Autodesk Fusion 360 part; units mm, degrees
note: some values were not read from the file. Set by a fixed rule: which sketch regions a step uses.
(part 26 of 59)
  spline S30 degree 5 poles (-12.6495, -13.6461) (-12.6495, -13.6462) (-12.6496, -13.6464) (-12.6497, -13.6467) (-12.65, -13.6471) (-12.6503, -13.6478) (-12.6506, -13.6486) (-12.651, -13.6495) (-12.6515, -13.6504) (-12.652, -13.6515) (-12.6526, -13.6527) (-12.6531, -13.654) (-12.6538, -13.6554) (-12.6544, -13.6569) (-12.6551, -13.6585) (-12.6559, -13.6602) (-12.6567, -13.6619) (-12.6575, -13.6638) (-12.6583, -13.6658) (-12.6592, -13.6678) (-12.6602, -13.67) (-12.6611, -13.6722) (-12.6621, -13.6745) (-12.6631, -13.6769) (-12.6642, -13.6794) (-12.6653, -13.682) (-12.6664, -13.6847) (-12.6676, -13.6874) (-12.6687, -13.6903) (-12.6699, -13.6932) (-12.6712, -13.6962) (-12.6724, -13.6993) (-12.6737, -13.7024) (-12.675, -13.7057) (-12.6764, -13.709) (-12.6778, -13.7124) (-12.6791, -13.7159) (-12.6806, -13.7195) (-12.682, -13.7231) (-12.6834, -13.7269) (-12.6849, -13.7307) (-12.6864, -13.7345) (-12.688, -13.7385) (-12.6895, -13.7425) (-12.6911, -13.7466) (-12.6927, -13.7508) (-12.6943, -13.755) (-12.6959, -13.7594) (-12.6975, -13.7638) (-12.6992, -13.7682) (-12.7009, -13.7728) (-12.7026, -13.7774) (-12.7043, -13.782) (-12.706, -13.7868) (-12.7077, -13.7916) (-12.7095, -13.7965) (-12.7113, -13.8015) (-12.7131, -13.8065) (-12.7149, -13.8116) (-12.7167, -13.8167) (-12.7185, -13.822) (-12.7204, -13.8273) (-12.7222, -13.8326) (-12.7241, -13.838) (-12.726, -13.8435) (-12.7279, -13.8491) (-12.7298, -13.8547) (-12.7317, -13.8604) (-12.7336, -13.8661) (-12.7356, -13.8719) (-12.7375, -13.8778) (-12.7395, -13.8837) (-12.7414, -13.8897) (-12.7434, -13.8958) (-12.7454, -13.9019) (-12.7474, -13.9081) (-12.7494, -13.9144) (-12.7514, -13.9207) (-12.7534, -13.927) (-12.7555, -13.9335) (-12.7575, -13.9399) (-12.7596, -13.9465) (-12.7616, -13.9531) (-12.7637, -13.9598) (-12.7657, -13.9665) (-12.7678, -13.9733) (-12.7699, -13.9801) (-12.772, -13.987) (-12.774, -13.9939) (-12.7761, -14.0009) (-12.7782, -14.008) (-12.7803, -14.0151) (-12.7824, -14.0223) (-12.7845, -14.0296) (-12.7867, -14.0368) (-12.7888, -14.0442) (-12.7909, -14.0516) (-12.793, -14.059) (-12.7952, -14.0665) (-12.7973, -14.0741) (-12.7994, -14.0817) (-12.8016, -14.0894) (-12.8037, -14.0971) (-12.8058, -14.1049) (-12.808, -14.1127) (-12.8101, -14.1206) (-12.8123, -14.1286) (-12.8144, -14.1365) (-12.8166, -14.1446) (-12.8187, -14.1527) (-12.8208, -14.1608) (-12.823, -14.169) (-12.8251, -14.1773) (-12.8273, -14.1856) (-12.8294, -14.1939) (-12.8316, -14.2023) (-12.8337, -14.2108) (-12.8359, -14.2193) (-12.838, -14.2278) (-12.8402, -14.2364) (-12.8423, -14.2451) (-12.8445, -14.2537) (-12.8466, -14.2625) (-12.8487, -14.2713) (-12.8509, -14.2801) (-12.853, -14.289) (-12.8551, -14.298) (-12.8573, -14.3069) (-12.8594, -14.316) (-12.8615, -14.3251) (-12.8636, -14.3342) (-12.8658, -14.3434) (-12.8679, -14.3526) (-12.87, -14.3619) (-12.8721, -14.3712) (-12.8742, -14.3806) (-12.8763, -14.39) (-12.8784, -14.3994) (-12.8805, -14.4089) (-12.8826, -14.4185) (-12.8847, -14.4281) (-12.8867, -14.4377) (-12.8888, -14.4474) (-12.8909, -14.4571) (-12.8929, -14.4669) (-12.895, -14.4767) (-12.8971, -14.4866) (-12.8991, -14.4965) (-12.9011, -14.5064) (-12.9032, -14.5164) (-12.9052, -14.5265) (-12.9072, -14.5365) (-12.9093, -14.5467) (-12.9113, -14.5568) (-12.9133, -14.5671) (-12.9153, -14.5773) (-12.9173, -14.5876) (-12.9193, -14.5979) (-12.9213, -14.6083) (-12.9232, -14.6188) (-12.9252, -14.6292) (-12.9272, -14.6397) (-12.9291, -14.6503) (-12.9311, -14.6609) (-12.933, -14.6715) (-12.9349, -14.6822) (-12.9368, -14.6929) (-12.9388, -14.7037) (-12.9407, -14.7145) (-12.9426, -14.7253) (-12.9445, -14.7362) (-12.9463, -14.7471) (-12.9482, -14.7581) (-12.9501, -14.7691) (-12.9519, -14.7801) (-12.9538, -14.7912) (-12.9556, -14.8023) (-12.9574, -14.8135) (-12.9593, -14.8247) (-12.9611, -14.8359) (-12.9629, -14.8472) (-12.9647, -14.8585) (-12.9665, -14.8699) (-12.9682, -14.8813) (-12.97, -14.8927) (-12.9718, -14.9042) (-12.9735, -14.9157) (-12.9752, -14.9273) (-12.977, -14.9388) (-12.9787, -14.9505) (-12.9804, -14.9621) (-12.9821, -14.9738) (-12.9838, -14.9856) (-12.9854, -14.9974) (-12.9871, -15.0092) (-12.9887, -15.021) (-12.9904, -15.0329) (-12.992, -15.0449) (-12.9936, -15.0568) (-12.9952, -15.0688) (-12.9968, -15.0809) (-12.9984, -15.0929) (-13, -15.105) (-13.0016, -15.1172) (-13.0031, -15.1294) (-13.0047, -15.1416) (-13.0062, -15.1539) (-13.0077, -15.1661) (-13.0092, -15.1785) (-13.0107, -15.1908) (-13.0122, -15.2032) (-13.0136, -15.2157) (-13.0151, -15.2281) (-13.0165, -15.2406) (-13.018, -15.2532) (-13.0194, -15.2658) (-13.0208, -15.2784) (-13.0222, -15.291) (-13.0236, -15.3037) (-13.0249, -15.3164) (-13.0263, -15.3291) (-13.0276, -15.3419) (-13.029, -15.3547) (-13.0303, -15.3676) (-13.0316, -15.3805) (-13.0329, -15.3934) (-13.0342, -15.4063) (-13.0354, -15.4193) (-13.0367, -15.4323) (-13.0379, -15.4454) (-13.0391, -15.4585) (-13.0404, -15.4716) (-13.0415, -15.4848) (-13.0427, -15.4979) (-13.0439, -15.5112) (-13.0451, -15.5244) (-13.0462, -15.5377) (-13.0473, -15.551) (-13.0484, -15.5644) (-13.0495, -15.5777) (-13.0506, -15.5911) (-13.0515, -15.6019) (-13.0521, -15.61) (-13.0525, -15.6154) (-13.0527, -15.6181) knots 0 0 0 0 0 0 0.00416667 0.00833333 0.0125 0.01666667 0.02083333 0.025 0.02916667 0.03333333 0.0375 0.04166667 0.04583333 0.05 0.05416667 0.05833333 0.0625 0.06666667 0.07083333 0.075 0.07916667 0.08333333 0.0875 0.09166667 0.09583333 0.1 0.10416667 0.10833333 0.1125 0.11666667 0.12083333 0.125 0.12916667 0.13333333 0.1375 0.14166667 0.14583333 0.15 0.15416667 0.15833333 0.1625 0.16666667 0.17083333 0.175 0.17916667 0.18333333 0.1875 0.19166667 0.19583333 0.2 0.20416667 0.20833333 0.2125 0.21666667 0.22083333 0.225 0.22916667 0.23333333 0.2375 0.24166667 0.24583333 0.25 0.25416667 0.25833333 0.2625 0.26666667 0.27083333 0.275 0.27916667 0.28333333 0.2875 0.29166667 0.29583333 0.3 0.30416667 0.30833333 0.3125 0.31666667 0.32083333 0.325 0.32916667 0.33333333 0.3375 0.34166667 0.34583333 0.35 0.35416667 0.35833333 0.3625 0.36666667 0.37083333 0.375 0.37916667 0.38333333 0.3875 0.39166667 0.39583333 0.4 0.40416667 0.40833333 0.4125 0.41666667 0.42083333 0.425 0.42916667 0.43333333 0.4375 0.44166667 0.44583333 0.45 0.45416667 0.45833333 0.4625 0.46666667 0.47083333 0.475 0.47916667 0.48333333 0.4875 0.49166667 0.49583333 0.5 0.50416667 0.50833333 0.5125 0.51666667 0.52083333 0.525 0.52916667 0.53333333 0.5375 0.54166667 0.54583333 0.55 0.55416667 0.55833333 0.5625 0.56666667 0.57083333 0.575 0.57916667 0.58333333 0.5875 0.59166667 0.59583333 0.6 0.60416667 0.60833333 0.6125 0.61666667 0.62083333 0.625 0.62916667 0.63333333 0.6375 0.64166667 0.64583333 0.65 0.65416667 0.65833333 0.6625 0.66666667 0.67083333 0.675 0.67916667 0.68333333 0.6875 0.69166667 0.69583333 0.7 0.70416667 0.70833333 0.7125 0.71666667 0.72083333 0.725 0.72916667 0.73333333 0.7375 0.74166667 0.74583333 0.75 0.75416667 0.75833333 0.7625 0.76666667 0.77083333 0.775 0.77916667 0.78333333 0.7875 0.79166667 0.79583333 0.8 0.80416667 0.80833333 0.8125 0.81666667 0.82083333 0.825 0.82916667 0.83333333 0.8375 0.84166667 0.84583333 0.85 0.85416667 0.85833333 0.8625 0.86666667 0.87083333 0.875 0.87916667 0.88333333 0.8875 0.89166667 0.89583333 0.9 0.90416667 0.90833333 0.9125 0.91666667 0.92083333 0.925 0.92916667 0.93333333 0.9375 0.94166667 0.94583333 0.95 0.95416667 0.95833333 0.9625 0.96666667 0.97083333 0.975 0.97916667 0.98333333 0.9875 0.99166667 0.99583333 1 1 1 1 1 1
  arc A39 (-13.0527, -15.6181) -> (-12.1618, -16.0147) centre (0, 12.5) ccw
  spline S31 degree 5 poles (-12.1618, -16.0147) (-12.16, -16.0128) (-12.1562, -16.0089) (-12.1506, -16.003) (-12.1432, -15.9951) (-12.134, -15.9854) (-12.1248, -15.9756) (-12.1156, -15.9658) (-12.1065, -15.9561) (-12.0973, -15.9464) (-12.0883, -15.9366) (-12.0792, -15.9269) (-12.0702, -15.9172) (-12.0613, -15.9075) (-12.0523, -15.8978) (-12.0434, -15.8882) (-12.0345, -15.8785) (-12.0257, -15.8689) (-12.0169, -15.8593) (-12.0081, -15.8496) (-11.9994, -15.84) (-11.9907, -15.8305) (-11.982, -15.8209) (-11.9734, -15.8113) (-11.9648, -15.8018) (-11.9562, -15.7922) (-11.9477, -15.7827) (-11.9392, -15.7732) (-11.9307, -15.7637) (-11.9223, -15.7542) (-11.9139, -15.7447) (-11.9055, -15.7353) (-11.8972, -15.7259) (-11.8889, -15.7164) (-11.8807, -15.707) (-11.8724, -15.6976) (-11.8643, -15.6882) (-11.8561, -15.6789) (-11.848, -15.6695) (-11.8399, -15.6602) (-11.8318, -15.6509) (-11.8238, -15.6416) (-11.8158, -15.6323) (-11.8079, -15.623) (-11.8, -15.6137) (-11.7921, -15.6045) (-11.7843, -15.5953) (-11.7765, -15.5861) (-11.7687, -15.5769) (-11.7609, -15.5677) (-11.7532, -15.5585) (-11.7456, -15.5494) (-11.7379, -15.5403) (-11.7303, -15.5312) (-11.7228, -15.5221) (-11.7153, -15.513) (-11.7078, -15.5039) (-11.7003, -15.4949) (-11.6929, -15.4859) (-11.6855, -15.4769) (-11.6781, -15.4679) (-11.6708, -15.4589) (-11.6635, -15.45) (-11.6563, -15.4411) (-11.6491, -15.4322) (-11.6419, -15.4233) (-11.6348, -15.4144) (-11.6276, -15.4055) (-11.6206, -15.3967) (-11.6135, -15.3879) (-11.6065, -15.3791) (-11.5996, -15.3704) (-11.5927, -15.3616) (-11.5858, -15.3529) (-11.5789, -15.3442) (-11.5721, -15.3355) (-11.5653, -15.3268) (-11.5585, -15.3182) (-11.5518, -15.3096) (-11.5452, -15.301) (-11.5385, -15.2924) (-11.5319, -15.2838) (-11.5253, -15.2753) (-11.5188, -15.2668) (-11.5123, -15.2583) (-11.5058, -15.2498) (-11.4994, -15.2414) (-11.493, -15.233) (-11.4867, -15.2246) (-11.4803, -15.2162) (-11.4741, -15.2078) (-11.4678, -15.1995) (-11.4616, -15.1912) (-11.4554, -15.1829) (-11.4493, -15.1747) (-11.4432, -15.1665) (-11.4371, -15.1582) (-11.4311, -15.1501) (-11.4251, -15.1419) (-11.4192, -15.1338) (-11.4132, -15.1257) (-11.4074, -15.1176) (-11.4015, -15.1096) (-11.3957, -15.1015) (-11.3899, -15.0936) (-11.3842, -15.0856) (-11.3785, -15.0776) (-11.3728, -15.0697) (-11.3672, -15.0618) (-11.3616, -15.054) (-11.3561, -15.0462) (-11.3506, -15.0384) (-11.3451, -15.0306) (-11.3396, -15.0228) (-11.3342, -15.0151) (-11.3289, -15.0074) (-11.3235, -14.9998) (-11.3183, -14.9922) (-11.313, -14.9846) (-11.3078, -14.977) (-11.3026, -14.9695) (-11.2975, -14.962) (-11.2924, -14.9545) (-11.2873, -14.947) (-11.2823, -14.9396) (-11.2773, -14.9323) (-11.2723, -14.9249) (-11.2674, -14.9176) (-11.2625, -14.9103) (-11.2577, -14.9031) (-11.2529, -14.8958) (-11.2481, -14.8887) (-11.2434, -14.8815) (-11.2387, -14.8744) (-11.234, -14.8673) (-11.2294, -14.8603) (-11.2248, -14.8533) (-11.2203, -14.8463) (-11.2158, -14.8393) (-11.2113, -14.8324) (-11.2069, -14.8256) (-11.2025, -14.8187) (-11.1982, -14.8119) (-11.1939, -14.8052) (-11.1896, -14.7985) (-11.1854, -14.7918) (-11.1812, -14.7851) (-11.177, -14.7785) (-11.1729, -14.772) (-11.1688, -14.7654) (-11.1648, -14.759) (-11.1608, -14.7525) (-11.1568, -14.7461) (-11.1529, -14.7397) (-11.149, -14.7334) (-11.1451, -14.7271) (-11.1413, -14.7209) (-11.1376, -14.7147) (-11.1338, -14.7085) (-11.1301, -14.7024) (-11.1265, -14.6963) (-11.1229, -14.6903) (-11.1193, -14.6843) (-11.1158, -14.6784) (-11.1123, -14.6725) (-11.1088, -14.6666) (-11.1054, -14.6608) (-11.102, -14.655) (-11.0987, -14.6493) (-11.0954, -14.6436) (-11.0921, -14.638) (-11.0889, -14.6324) (-11.0857, -14.6269) (-11.0826, -14.6214) (-11.0795, -14.616) (-11.0764, -14.6106) (-11.0734, -14.6053) (-11.0704, -14.6) (-11.0675, -14.5948) (-11.0646, -14.5896) (-11.0617, -14.5845) (-11.0589, -14.5794) (-11.0561, -14.5744) (-11.0534, -14.5694) (-11.0507, -14.5645) (-11.048, -14.5597) (-11.0454, -14.5549) (-11.0428, -14.5501) (-11.0403, -14.5454) (-11.0378, -14.5408) (-11.0353, -14.5362) (-11.0329, -14.5317) (-11.0306, -14.5272) (-11.0282, -14.5228) (-11.0259, -14.5185) (-11.0237, -14.5142) (-11.0215, -14.51) (-11.0193, -14.5058) (-11.0172, -14.5017) (-11.0151, -14.4977) (-11.0131, -14.4937) (-11.0111, -14.4898) (-11.0091, -14.486) (-11.0072, -14.4822) (-11.0053, -14.4785) (-11.0035, -14.4748) (-11.0017, -14.4713) (-10.9999, -14.4678) (-10.9982, -14.4643) (-10.9966, -14.461) (-10.9949, -14.4577) (-10.9934, -14.4544) (-10.9918, -14.4513) (-10.9903, -14.4482) (-10.9889, -14.4452) (-10.9875, -14.4423) (-10.9861, -14.4394) (-10.9848, -14.4366) (-10.9835, -14.4339) (-10.9823, -14.4313) (-10.9811, -14.4288) (-10.9799, -14.4263) (-10.9788, -14.424) (-10.9778, -14.4217) (-10.9768, -14.4195) (-10.9758, -14.4173) (-10.9749, -14.4153) (-10.974, -14.4134) (-10.9731, -14.4115) (-10.9724, -14.4097) (-10.9716, -14.408) (-10.9709, -14.4065) (-10.9702, -14.405) (-10.9696, -14.4036) (-10.9691, -14.4023) (-10.9685, -14.4011) (-10.9681, -14.4) (-10.9676, -14.399) (-10.9672, -14.3981) (-10.9669, -14.3973) (-10.9666, -14.3966) (-10.9664, -14.3961) (-10.9663, -14.3958) (-10.9662, -14.3956) (-10.9662, -14.3955) knots -1 -1 -1 -1 -1 -1 -0.99583333 -0.99166667 -0.9875 -0.98333333 -0.97916667 -0.975 -0.97083333 -0.96666667 -0.9625 -0.95833333 -0.95416667 -0.95 -0.94583333 -0.94166667 -0.9375 -0.93333333 -0.92916667 -0.925 -0.92083333 -0.91666667 -0.9125 -0.90833333 -0.90416667 -0.9 -0.89583333 -0.89166667 -0.8875 -0.88333333 -0.87916667 -0.875 -0.87083333 -0.86666667 -0.8625 -0.85833333 -0.85416667 -0.85 -0.84583333 -0.84166667 -0.8375 -0.83333333 -0.82916667 -0.825 -0.82083333 -0.81666667 -0.8125 -0.80833333 -0.80416667 -0.8 -0.79583333 -0.79166667 -0.7875 -0.78333333 -0.77916667 -0.775 -0.77083333 -0.76666667 -0.7625 -0.75833333 -0.75416667 -0.75 -0.74583333 -0.74166667 -0.7375 -0.73333333 -0.72916667 -0.725 -0.72083333 -0.71666667 -0.7125 -0.70833333 -0.70416667 -0.7 -0.69583333 -0.69166667 -0.6875 -0.68333333 -0.67916667 -0.675 -0.67083333 -0.66666667 -0.6625 -0.65833333 -0.65416667 -0.65 -0.64583333 -0.64166667 -0.6375 -0.63333333 -0.62916667 -0.625 -0.62083333 -0.61666667 -0.6125 -0.60833333 -0.60416667 -0.6 -0.59583333 -0.59166667 -0.5875 -0.58333333 -0.57916667 -0.575 -0.57083333 -0.56666667 -0.5625 -0.55833333 -0.55416667 -0.55 -0.54583333 -0.54166667 -0.5375 -0.53333333 -0.52916667 -0.525 -0.52083333 -0.51666667 -0.5125 -0.50833333 -0.50416667 -0.5 -0.49583333 -0.49166667 -0.4875 -0.48333333 -0.47916667 -0.475 -0.47083333 -0.46666667 -0.4625 -0.45833333 -0.45416667 -0.45 -0.44583333 -0.44166667 -0.4375 -0.43333333 -0.42916667 -0.425 -0.42083333 -0.41666667 -0.4125 -0.40833333 -0.40416667 -0.4 -0.39583333 -0.39166667 -0.3875 -0.38333333 -0.37916667 -0.375 -0.37083333 -0.36666667 -0.3625 -0.35833333 -0.35416667 -0.35 -0.34583333 -0.34166667 -0.3375 -0.33333333 -0.32916667 -0.325 -0.32083333 -0.31666667 -0.3125 -0.30833333 -0.30416667 -0.3 -0.29583333 -0.29166667 -0.2875 -0.28333333 -0.27916667 -0.275 -0.27083333 -0.26666667 -0.2625 -0.25833333 -0.25416667 -0.25 -0.24583333 -0.24166667 -0.2375 -0.23333333 -0.22916667 -0.225 -0.22083333 -0.21666667 -0.2125 -0.20833333 -0.20416667 -0.2 -0.19583333 -0.19166667 -0.1875 -0.18333333 -0.17916667 -0.175 -0.17083333 -0.16666667 -0.1625 -0.15833333 -0.15416667 -0.15 -0.14583333 -0.14166667 -0.1375 -0.13333333 -0.12916667 -0.125 -0.12083333 -0.11666667 -0.1125 -0.10833333 -0.10416667 -0.1 -0.09583333 -0.09166667 -0.0875 -0.08333333 -0.07916667 -0.075 -0.07083333 -0.06666667 -0.0625 -0.05833333 -0.05416667 -0.05 -0.04583333 -0.04166667 -0.0375 -0.03333333 -0.02916667 -0.025 -0.02083333 -0.01666667 -0.0125 -0.00833333 -0.00416667 0 0 0 0 0 0
  line L63 (-10.9662, -14.3955) -> (-10.9659, -14.3948)
  line L64 (-10.9659, -14.3948) -> (-10.8547, -14.1221)
  arc A40 (-10.8547, -14.1221) -> (-9.7471, -14.5473) centre (0, 12.5) ccw
  line L65 (-9.7471, -14.5473) -> (-9.8469, -14.8243)
  line L66 (-9.8469, -14.8243) -> (-9.8472, -14.8251)
  spline S32 degree 5 poles (-9.8472, -14.8251) (-9.8472, -14.8252) (-9.8473, -14.8254) (-9.8474, -14.8257) (-9.8475, -14.8262) (-9.8478, -14.8269) (-9.8481, -14.8277) (-9.8484, -14.8286) (-9.8487, -14.8296) (-9.8491, -14.8308) (-9.8495, -14.832) (-9.85, -14.8334) (-9.8505, -14.8348) (-9.851, -14.8364) (-9.8515, -14.838) (-9.8521, -14.8398) (-9.8527, -14.8416) (-9.8533, -14.8435) (-9.8539, -14.8456) (-9.8546, -14.8477) (-9.8553, -14.8499) (-9.856, -14.8523) (-9.8568, -14.8547) (-9.8575, -14.8572) (-9.8583, -14.8598) (-9.8591, -14.8625) (-9.86, -14.8652) (-9.8608, -14.8681) (-9.8617, -14.871) (-9.8626, -14.8741) (-9.8635, -14.8772) (-9.8645, -14.8804) (-9.8654, -14.8837) (-9.8664, -14.887) (-9.8674, -14.8905) (-9.8684, -14.894) (-9.8694, -14.8976) (-9.8704, -14.9013) (-9.8715, -14.9051) (-9.8725, -14.909) (-9.8736, -14.9129) (-9.8747, -14.9169) (-9.8758, -14.921) (-9.8769, -14.9252) (-9.878, -14.9294) (-9.8792, -14.9337) (-9.8803, -14.9381) (-9.8815, -14.9426) (-9.8827, -14.9471) (-9.8838, -14.9517) (-9.885, -14.9564) (-9.8862, -14.9612) (-9.8874, -14.966) (-9.8887, -14.9709) (-9.8899, -14.9759) (-9.8911, -14.981) (-9.8924, -14.9861) (-9.8936, -14.9912) (-9.8949, -14.9965) (-9.8962, -15.0018) (-9.8974, -15.0072) (-9.8987, -15.0127) (-9.9, -15.0182) (-9.9013, -15.0238) (-9.9026, -15.0294) (-9.9039, -15.0352) (-9.9052, -15.0409) (-9.9065, -15.0468) (-9.9079, -15.0527) (-9.9092, -15.0587) (-9.9105, -15.0647) (-9.9118, -15.0709) (-9.9132, -15.077) (-9.9145, -15.0833) (-9.9158, -15.0896) (-9.9172, -15.0959) (-9.9185, -15.1023) (-9.9199, -15.1088) (-9.9212, -15.1154) (-9.9225, -15.122) (-9.9239, -15.1286) (-9.9252, -15.1353) (-9.9266, -15.1421) (-9.9279, -15.149) (-9.9293, -15.1559) (-9.9306, -15.1628) (-9.932, -15.1698) (-9.9333, -15.1769) (-9.9347, -15.1841) (-9.936, -15.1912) (-9.9374, -15.1985) (-9.9387, -15.2058) (-9.9401, -15.2132) (-9.9414, -15.2206) (-9.9428, -15.228) (-9.9441, -15.2356) (-9.9454, -15.2431) (-9.9468, -15.2508) (-9.9481, -15.2585) (-9.9494, -15.2662) (-9.9508, -15.274) (-9.9521, -15.2819) (-9.9534, -15.2898) (-9.9547, -15.2977) (-9.956, -15.3057) (-9.9573, -15.3138) (-9.9586, -15.3219) (-9.9599, -15.3301) (-9.9612, -15.3383) (-9.9625, -15.3466) (-9.9638, -15.3549) (-9.9651, -15.3633) (-9.9664, -15.3717) (-9.9676, -15.3802) (-9.9689, -15.3887) (-9.9701, -15.3973) (-9.9714, -15.4059) (-9.9726, -15.4146) (-9.9739, -15.4233) (-9.9751, -15.4321) (-9.9763, -15.4409) (-9.9776, -15.4498) (-9.9788, -15.4587) (-9.98, -15.4677) (-9.9812, -15.4767) (-9.9824, -15.4858) (-9.9836, -15.4949) (-9.9847, -15.504) (-9.9859, -15.5133) (-9.9871, -15.5225) (-9.9882, -15.5318) (-9.9894, -15.5412) (-9.9905, -15.5506) (-9.9916, -15.56) (-9.9928, -15.5695) (-9.9939, -15.579) (-9.995, -15.5886) (-9.9961, -15.5982) (-9.9972, -15.6079) (-9.9983, -15.6176) (-9.9993, -15.6274) (-10.0004, -15.6372) (-10.0014, -15.647) (-10.0025, -15.6569) (-10.0035, -15.6668) (-10.0045, -15.6768) (-10.0055, -15.6868) (-10.0065, -15.6969) (-10.0075, -15.707) (-10.0085, -15.7172) (-10.0095, -15.7274) (-10.0104, -15.7376) (-10.0114, -15.7479) (-10.0123, -15.7582) (-10.0133, -15.7686) (-10.0142, -15.779) (-10.0151, -15.7894) (-10.016, -15.7999) (-10.0169, -15.8105) (-10.0177, -15.821) (-10.0186, -15.8317) (-10.0195, -15.8423) (-10.0203, -15.853) (-10.0211, -15.8638) (-10.0219, -15.8745) (-10.0227, -15.8854) (-10.0235, -15.8962) (-10.0243, -15.9071) (-10.0251, -15.9181) (-10.0258, -15.929) (-10.0266, -15.94) (-10.0273, -15.9511) (-10.028, -15.9622) (-10.0287, -15.9733) (-10.0294, -15.9845) (-10.0301, -15.9957) (-10.0308, -16.007) (-10.0314, -16.0183) (-10.0321, -16.0296) (-10.0327, -16.041) (-10.0333, -16.0524) (-10.0339, -16.0638) (-10.0345, -16.0753) (-10.0351, -16.0868) (-10.0356, -16.0984) (-10.0362, -16.11) (-10.0367, -16.1216) (-10.0372, -16.1333) (-10.0377, -16.145) (-10.0382, -16.1567) (-10.0387, -16.1685) (-10.0392, -16.1803) (-10.0396, -16.1922) (-10.04, -16.2041) (-10.0405, -16.216) (-10.0409, -16.228) (-10.0412, -16.24) (-10.0416, -16.252) (-10.042, -16.2641) (-10.0423, -16.2762) (-10.0427, -16.2883) (-10.043, -16.3005) (-10.0433, -16.3127) (-10.0436, -16.3249) (-10.0438, -16.3372) (-10.0441, -16.3495) (-10.0443, -16.3619) (-10.0445, -16.3743) (-10.0448, -16.3867) (-10.0449, -16.3991) (-10.0451, -16.4116) (-10.0453, -16.4241) (-10.0454, -16.4367) (-10.0456, -16.4493) (-10.0457, -16.4619) (-10.0458, -16.4745) (-10.0458, -16.4872) (-10.0459, -16.5) (-10.046, -16.5127) (-10.046, -16.5255) (-10.046, -16.5383) (-10.046, -16.5512) (-10.046, -16.5641) (-10.046, -16.577) (-10.0459, -16.5899) (-10.0458, -16.6029) (-10.0458, -16.6159) (-10.0457, -16.629) (-10.0455, -16.642) (-10.0454, -16.6551) (-10.0453, -16.6683) (-10.0451, -16.6815) (-10.0449, -16.6947) (-10.0447, -16.7079) (-10.0445, -16.7212) (-10.0442, -16.7345) (-10.044, -16.7478) (-10.0437, -16.7612) (-10.0434, -16.7745) (-10.0431, -16.788) (-10.0428, -16.8014) (-10.0425, -16.8122) (-10.0423, -16.8203) (-10.0422, -16.8257) (-10.0421, -16.8284) knots 0 0 0 0 0 0 0.00416667 0.00833333 0.0125 0.01666667 0.02083333 0.025 0.02916667 0.03333333 0.0375 0.04166667 0.04583333 0.05 0.05416667 0.05833333 0.0625 0.06666667 0.07083333 0.075 0.07916667 0.08333333 0.0875 0.09166667 0.09583333 0.1 0.10416667 0.10833333 0.1125 0.11666667 0.12083333 0.125 0.12916667 0.13333333 0.1375 0.14166667 0.14583333 0.15 0.15416667 0.15833333 0.1625 0.16666667 0.17083333 0.175 0.17916667 0.18333333 0.1875 0.19166667 0.19583333 0.2 0.20416667 0.20833333 0.2125 0.21666667 0.22083333 0.225 0.22916667 0.23333333 0.2375 0.24166667 0.24583333 0.25 0.25416667 0.25833333 0.2625 0.26666667 0.27083333 0.275 0.27916667 0.28333333 0.2875 0.29166667 0.29583333 0.3 0.30416667 0.30833333 0.3125 0.31666667 0.32083333 0.325 0.32916667 0.33333333 0.3375 0.34166667 0.34583333 0.35 0.35416667 0.35833333 0.3625 0.36666667 0.37083333 0.375 0.37916667 0.38333333 0.3875 0.39166667 0.39583333 0.4 0.40416667 0.40833333 0.4125 0.41666667 0.42083333 0.425 0.42916667 0.43333333 0.4375 0.44166667 0.44583333 0.45 0.45416667 0.45833333 0.4625 0.46666667 0.47083333 0.475 0.47916667 0.48333333 0.4875 0.49166667 0.49583333 0.5 0.50416667 0.50833333 0.5125 0.51666667 0.52083333 0.525 0.52916667 0.53333333 0.5375 0.54166667 0.54583333 0.55 0.55416667 0.55833333 0.5625 0.56666667 0.57083333 0.575 0.57916667 0.58333333 0.5875 0.59166667 0.59583333 0.6 0.60416667 0.60833333 0.6125 0.61666667 0.62083333 0.625 0.62916667 0.63333333 0.6375 0.64166667 0.64583333 0.65 0.65416667 0.65833333 0.6625 0.66666667 0.67083333 0.675 0.67916667 0.68333333 0.6875 0.69166667 0.69583333 0.7 0.70416667 0.70833333 0.7125 0.71666667 0.72083333 0.725 0.72916667 0.73333333 0.7375 0.74166667 0.74583333 0.75 0.75416667 0.75833333 0.7625 0.76666667 0.77083333 0.775 0.77916667 0.78333333 0.7875 0.79166667 0.79583333 0.8 0.80416667 0.80833333 0.8125 0.81666667 0.82083333 0.825 0.82916667 0.83333333 0.8375 0.84166667 0.84583333 0.85 0.85416667 0.85833333 0.8625 0.86666667 0.87083333 0.875 0.87916667 0.88333333 0.8875 0.89166667 0.89583333 0.9 0.90416667 0.90833333 0.9125 0.91666667 0.92083333 0.925 0.92916667 0.93333333 0.9375 0.94166667 0.94583333 0.95 0.95416667 0.95833333 0.9625 0.96666667 0.97083333 0.975 0.97916667 0.98333333 0.9875 0.99166667 0.99583333 1 1 1 1 1 1
  arc A41 (-10.0421, -16.8284) -> (-9.1146, -17.1298) centre (0, 12.5) ccw
  spline S33 degree 5 poles (-9.1146, -17.1298) (-9.1129, -17.1276) (-9.1096, -17.1234) (-9.1047, -17.1169) (-9.0981, -17.1084) (-9.09, -17.0977) (-9.0818, -17.087) (-9.0737, -17.0763) (-9.0657, -17.0657) (-9.0576, -17.055) (-9.0496, -17.0444) (-9.0416, -17.0338) (-9.0337, -17.0232) (-9.0258, -17.0127) (-9.0179, -17.0021) (-9.0101, -16.9915) (-9.0022, -16.981) (-8.9945, -16.9705) (-8.9867, -16.96) (-8.979, -16.9495) (-8.9713, -16.9391) (-8.9637, -16.9286) (-8.956, -16.9182) (-8.9485, -16.9078) (-8.9409, -16.8974) (-8.9334, -16.887) (-8.9259, -16.8766) (-8.9184, -16.8663) (-8.911, -16.856) (-8.9036, -16.8457) (-8.8963, -16.8354) (-8.8889, -16.8251) (-8.8816, -16.8148) (-8.8744, -16.8046) (-8.8671, -16.7944) (-8.86, -16.7842) (-8.8528, -16.774) (-8.8457, -16.7638) (-8.8386, -16.7537) (-8.8315, -16.7435) (-8.8245, -16.7334) (-8.8175, -16.7233) (-8.8105, -16.7132) (-8.8036, -16.7032) (-8.7967, -16.6932) (-8.7898, -16.6831) (-8.783, -16.6731) (-8.7762, -16.6632) (-8.7694, -16.6532) (-8.7626, -16.6433) (-8.7559, -16.6334) (-8.7493, -16.6235) (-8.7426, -16.6136) (-8.736, -16.6037) (-8.7295, -16.5939) (-8.7229, -16.5841) (-8.7164, -16.5743) (-8.7099, -16.5646) (-8.7035, -16.5548) (-8.6971, -16.5451) (-8.6907, -16.5354) (-8.6844, -16.5257) (-8.6781, -16.516) (-8.6718, -16.5064) (-8.6656, -16.4968) (-8.6593, -16.4872) (-8.6532, -16.4776) (-8.647, -16.4681) (-8.6409, -16.4586) (-8.6348, -16.4491) (-8.6288, -16.4396) (-8.6228, -16.4302) (-8.6168, -16.4207) (-8.6109, -16.4113) (-8.605, -16.402) (-8.5991, -16.3926) (-8.5932, -16.3833) (-8.5874, -16.374) (-8.5817, -16.3647) (-8.5759, -16.3555) (-8.5702, -16.3462) (-8.5645, -16.337) (-8.5589, -16.3279) (-8.5533, -16.3187) (-8.5477, -16.3096) (-8.5422, -16.3005) (-8.5367, -16.2914) (-8.5312, -16.2824) (-8.5257, -16.2734) (-8.5203, -16.2644) (-8.515, -16.2554) (-8.5096, -16.2465) (-8.5043, -16.2376) (-8.499, -16.2287) (-8.4938, -16.2199) (-8.4886, -16.211) (-8.4834, -16.2022) (-8.4783, -16.1935) (-8.4732, -16.1847) (-8.4681, -16.176) (-8.463, -16.1674) (-8.458, -16.1587) (-8.4531, -16.1501) (-8.4481, -16.1415) (-8.4432, -16.133) (-8.4384, -16.1244) (-8.4335, -16.116) (-8.4287, -16.1075) (-8.4239, -16.0991) (-8.4192, -16.0907) (-8.4145, -16.0823) (-8.4098, -16.074) (-8.4052, -16.0657) (-8.4006, -16.0574) (-8.396, -16.0491) (-8.3915, -16.0409) (-8.387, -16.0328) (-8.3825, -16.0246) (-8.3781, -16.0165) (-8.3737, -16.0085) (-8.3693, -16.0004) (-8.365, -15.9924) (-8.3607, -15.9845) (-8.3565, -15.9765) (-8.3522, -15.9686) (-8.348, -15.9608) (-8.3439, -15.9529) (-8.3398, -15.9452) (-8.3357, -15.9374) (-8.3316, -15.9297) (-8.3276, -15.922) (-8.3236, -15.9144) (-8.3196, -15.9068) (-8.3157, -15.8992) (-8.3118, -15.8917) (-8.308, -15.8842) (-8.3042, -15.8767) (-8.3004, -15.8693) (-8.2966, -15.8619) (-8.2929, -15.8546) (-8.2892, -15.8473) (-8.2856, -15.8401) (-8.282, -15.8329) (-8.2784, -15.8257) (-8.2748, -15.8186) (-8.2713, -15.8115) (-8.2678, -15.8044) (-8.2644, -15.7974) (-8.261, -15.7905) (-8.2576, -15.7835) (-8.2543, -15.7767) (-8.251, -15.7698) (-8.2477, -15.763) (-8.2445, -15.7563) (-8.2412, -15.7496) (-8.2381, -15.7429) (-8.2349, -15.7363) (-8.2318, -15.7298) (-8.2288, -15.7233) (-8.2257, -15.7168) (-8.2227, -15.7104) (-8.2198, -15.704) (-8.2169, -15.6977) (-8.214, -15.6914) (-8.2111, -15.6851) (-8.2083, -15.679) (-8.2055, -15.6728) (-8.2027, -15.6667) (-8.2, -15.6607) (-8.1973, -15.6547) (-8.1947, -15.6488) (-8.192, -15.6429) (-8.1895, -15.6371) (-8.1869, -15.6313) (-8.1844, -15.6256) (-8.1819, -15.6199) (-8.1795, -15.6143) (-8.177, -15.6087) (-8.1747, -15.6032) (-8.1723, -15.5978) (-8.17, -15.5924) (-8.1677, -15.587) (-8.1655, -15.5818) (-8.1633, -15.5765) (-8.1611, -15.5714) (-8.159, -15.5663) (-8.1569, -15.5612) (-8.1548, -15.5562) (-8.1528, -15.5513) (-8.1508, -15.5464) (-8.1488, -15.5416) (-8.1469, -15.5369) (-8.145, -15.5322) (-8.1432, -15.5276) (-8.1413, -15.523) (-8.1395, -15.5185) (-8.1378, -15.5141) (-8.1361, -15.5097) (-8.1344, -15.5054) (-8.1327, -15.5012) (-8.1311, -15.497) (-8.1295, -15.4929) (-8.128, -15.4889) (-8.1265, -15.4849) (-8.125, -15.4811) (-8.1236, -15.4772) (-8.1222, -15.4735) (-8.1208, -15.4698) (-8.1194, -15.4662) (-8.1181, -15.4627) (-8.1169, -15.4593) (-8.1156, -15.4559) (-8.1144, -15.4526) (-8.1133, -15.4494) (-8.1121, -15.4462) (-8.1111, -15.4432) (-8.11, -15.4402) (-8.109, -15.4373) (-8.108, -15.4345) (-8.107, -15.4318) (-8.1061, -15.4291) (-8.1052, -15.4265) (-8.1044, -15.4241) (-8.1036, -15.4217) (-8.1028, -15.4194) (-8.102, -15.4172) (-8.1013, -15.415) (-8.1007, -15.413) (-8.1, -15.4111) (-8.0994, -15.4092) (-8.0988, -15.4075) (-8.0983, -15.4058) (-8.0978, -15.4043) (-8.0973, -15.4028) (-8.0969, -15.4015) (-8.0965, -15.4002) (-8.0962, -15.3991) (-8.0958, -15.398) (-8.0956, -15.3971) (-8.0953, -15.3963) (-8.0951, -15.3956) (-8.0949, -15.3951) (-8.0948, -15.3948) (-8.0948, -15.3946) (-8.0948, -15.3945) knots -1 -1 -1 -1 -1 -1 -0.99583333 -0.99166667 -0.9875 -0.98333333 -0.97916667 -0.975 -0.97083333 -0.96666667 -0.9625 -0.95833333 -0.95416667 -0.95 -0.94583333 -0.94166667 -0.9375 -0.93333333 -0.92916667 -0.925 -0.92083333 -0.91666667 -0.9125 -0.90833333 -0.90416667 -0.9 -0.89583333 -0.89166667 -0.8875 -0.88333333 -0.87916667 -0.875 -0.87083333 -0.86666667 -0.8625 -0.85833333 -0.85416667 -0.85 -0.84583333 -0.84166667 -0.8375 -0.83333333 -0.82916667 -0.825 -0.82083333 -0.81666667 -0.8125 -0.80833333 -0.80416667 -0.8 -0.79583333 -0.79166667 -0.7875 -0.78333333 -0.77916667 -0.775 -0.77083333 -0.76666667 -0.7625 -0.75833333 -0.75416667 -0.75 -0.74583333 -0.74166667 -0.7375 -0.73333333 -0.72916667 -0.725 -0.72083333 -0.71666667 -0.7125 -0.70833333 -0.70416667 -0.7 -0.69583333 -0.69166667 -0.6875 -0.68333333 -0.67916667 -0.675 -0.67083333 -0.66666667 -0.6625 -0.65833333 -0.65416667 -0.65 -0.64583333 -0.64166667 -0.6375 -0.63333333 -0.62916667 -0.625 -0.62083333 -0.61666667 -0.6125 -0.60833333 -0.60416667 -0.6 -0.59583333 -0.59166667 -0.5875 -0.58333333 -0.57916667 -0.575 -0.57083333 -0.56666667 -0.5625 -0.55833333 -0.55416667 -0.55 -0.54583333 -0.54166667 -0.5375 -0.53333333 -0.52916667 -0.525 -0.52083333 -0.51666667 -0.5125 -0.50833333 -0.50416667 -0.5 -0.49583333 -0.49166667 -0.4875 -0.48333333 -0.47916667 -0.475 -0.47083333 -0.46666667 -0.4625 -0.45833333 -0.45416667 -0.45 -0.44583333 -0.44166667 -0.4375 -0.43333333 -0.42916667 -0.425 -0.42083333 -0.41666667 -0.4125 -0.40833333 -0.40416667 -0.4 -0.39583333 -0.39166667 -0.3875 -0.38333333 -0.37916667 -0.375 -0.37083333 -0.36666667 -0.3625 -0.35833333 -0.35416667 -0.35 -0.34583333 -0.34166667 -0.3375 -0.33333333 -0.32916667 -0.325 -0.32083333 -0.31666667 -0.3125 -0.30833333 -0.30416667 -0.3 -0.29583333 -0.29166667 -0.2875 -0.28333333 -0.27916667 -0.275 -0.27083333 -0.26666667 -0.2625 -0.25833333 -0.25416667 -0.25 -0.24583333 -0.24166667 -0.2375 -0.23333333 -0.22916667 -0.225 -0.22083333 -0.21666667 -0.2125 -0.20833333 -0.20416667 -0.2 -0.19583333 -0.19166667 -0.1875 -0.18333333 -0.17916667 -0.175 -0.17083333 -0.16666667 -0.1625 -0.15833333 -0.15416667 -0.15 -0.14583333 -0.14166667 -0.1375 -0.13333333 -0.12916667 -0.125 -0.12083333 -0.11666667 -0.1125 -0.10833333 -0.10416667 -0.1 -0.09583333 -0.09166667 -0.0875 -0.08333333 -0.07916667 -0.075 -0.07083333 -0.06666667 -0.0625 -0.05833333 -0.05416667 -0.05 -0.04583333 -0.04166667 -0.0375 -0.03333333 -0.02916667 -0.025 -0.02083333 -0.01666667 -0.0125 -0.00833333 -0.00416667 0 0 0 0 0 0
  line L67 (-8.0948, -15.3945) -> (-8.0945, -15.3937)
  line L68 (-8.0945, -15.3937) -> (-8.0125, -15.1109)
  arc A42 (-8.0125, -15.1109) -> (-6.8665, -15.418) centre (0, 12.5) ccw
  line L69 (-6.8665, -15.418) -> (-6.9368, -15.7039)
  line L70 (-6.9368, -15.7039) -> (-6.937, -15.7047)
  spline S34 degree 5 poles (-6.937, -15.7047) (-6.937, -15.7048) (-6.937, -15.705) (-6.9371, -15.7053) (-6.9372, -15.7058) (-6.9374, -15.7065) (-6.9376, -15.7074) (-6.9378, -15.7083) (-6.9381, -15.7094) (-6.9383, -15.7106) (-6.9386, -15.7118) (-6.9389, -15.7132) (-6.9392, -15.7147) (-6.9396, -15.7163) (-6.9399, -15.718) (-6.9403, -15.7198) (-6.9407, -15.7217) (-6.9411, -15.7237) (-6.9416, -15.7258) (-6.942, -15.728) (-6.9425, -15.7303) (-6.9429, -15.7327) (-6.9434, -15.7351) (-6.9439, -15.7377) (-6.9445, -15.7404) (-6.945, -15.7431) (-6.9455, -15.746) (-6.9461, -15.7489) (-6.9466, -15.7519) (-6.9472, -15.755) (-6.9478, -15.7582) (-6.9484, -15.7615) (-6.949, -15.7649) (-6.9496, -15.7683) (-6.9502, -15.7719) (-6.9508, -15.7755) (-6.9515, -15.7792) (-6.9521, -15.783) (-6.9528, -15.7868) (-6.9534, -15.7908) (-6.9541, -15.7948) (-6.9547, -15.7989) (-6.9554, -15.8031) (-6.9561, -15.8074) (-6.9568, -15.8117) (-6.9574, -15.8161) (-6.9581, -15.8206) (-6.9588, -15.8252) (-6.9595, -15.8298) (-6.9602, -15.8345) (-6.9609, -15.8393) (-6.9616, -15.8442) (-6.9623, -15.8491) (-6.963, -15.8541) (-6.9637, -15.8592) (-6.9644, -15.8643) (-6.9651, -15.8695) (-6.9658, -15.8748) (-6.9665, -15.8802) (-6.9672, -15.8856) (-6.9679, -15.8911) (-6.9686, -15.8966) (-6.9693, -15.9023) (-6.97, -15.908) (-6.9707, -15.9137) (-6.9714, -15.9196) (-6.9721, -15.9255) (-6.9728, -15.9314) (-6.9735, -15.9374) (-6.9742, -15.9435) (-6.9749, -15.9497) (-6.9756, -15.9559) (-6.9763, -15.9622) (-6.9769, -15.9685) (-6.9776, -15.9749) (-6.9783, -15.9814) (-6.9789, -15.9879) (-6.9796, -15.9945) (-6.9803, -16.0011) (-6.9809, -16.0078) (-6.9816, -16.0146) (-6.9822, -16.0214) (-6.9828, -16.0283) (-6.9835, -16.0353) (-6.9841, -16.0423) (-6.9847, -16.0493) (-6.9853, -16.0564) (-6.9859, -16.0636) (-6.9865, -16.0709) (-6.9871, -16.0781) (-6.9877, -16.0855) (-6.9882, -16.0929) (-6.9888, -16.1004) (-6.9894, -16.1079) (-6.9899, -16.1154) (-6.9905, -16.1231) (-6.991, -16.1307) (-6.9915, -16.1385) (-6.9921, -16.1463) (-6.9926, -16.1541) (-6.9931, -16.162) (-6.9936, -16.17) (-6.994, -16.178) (-6.9945, -16.186) (-6.995, -16.1941) (-6.9954, -16.2023) (-6.9959, -16.2105) (-6.9963, -16.2187) (-6.9968, -16.227) (-6.9972, -16.2354) (-6.9976, -16.2438) (-6.998, -16.2523) (-6.9984, -16.2608) (-6.9987, -16.2694) (-6.9991, -16.278) (-6.9995, -16.2866) (-6.9998, -16.2953) (-7.0001, -16.3041) (-7.0005, -16.3129) (-7.0008, -16.3218) (-7.0011, -16.3307) (-7.0014, -16.3396) (-7.0016, -16.3486) (-7.0019, -16.3577) (-7.0021, -16.3668) (-7.0024, -16.3759) (-7.0026, -16.3851) (-7.0028, -16.3943) (-7.003, -16.4036) (-7.0032, -16.4129) (-7.0034, -16.4223) (-7.0036, -16.4317) (-7.0037, -16.4412) (-7.0038, -16.4507) (-7.004, -16.4602) (-7.0041, -16.4698) (-7.0042, -16.4795) (-7.0043, -16.4892) (-7.0043, -16.4989) (-7.0044, -16.5087) (-7.0044, -16.5185) (-7.0045, -16.5284) (-7.0045, -16.5383) (-7.0045, -16.5482) (-7.0045, -16.5582) (-7.0044, -16.5682) (-7.0044, -16.5783) (-7.0043, -16.5884) (-7.0043, -16.5986) (-7.0042, -16.6088) (-7.0041, -16.619) (-7.004, -16.6293) (-7.0038, -16.6396) (-7.0037, -16.65) (-7.0035, -16.6604) (-7.0034, -16.6708) (-7.0032, -16.6813) (-7.003, -16.6919) (-7.0028, -16.7024) (-7.0025, -16.713) (-7.0023, -16.7237) (-7.002, -16.7344) (-7.0017, -16.7451) (-7.0014, -16.7559) (-7.0011, -16.7667) (-7.0008, -16.7775) (-7.0004, -16.7884) (-7.0001, -16.7993) (-6.9997, -16.8103) (-6.9993, -16.8213) (-6.9989, -16.8323) (-6.9984, -16.8434) (-6.998, -16.8545) (-6.9975, -16.8657) (-6.997, -16.8768) (-6.9965, -16.8881) (-6.996, -16.8993) (-6.9955, -16.9106) (-6.995, -16.922) (-6.9944, -16.9333) (-6.9938, -16.9447) (-6.9932, -16.9562) (-6.9926, -16.9677) (-6.992, -16.9792) (-6.9913, -16.9907) (-6.9906, -17.0023) (-6.99, -17.014) (-6.9892, -17.0256) (-6.9885, -17.0373) (-6.9878, -17.049) (-6.987, -17.0608) (-6.9863, -17.0726) (-6.9855, -17.0844) (-6.9846, -17.0963) (-6.9838, -17.1082) (-6.983, -17.1201) (-6.9821, -17.1321) (-6.9812, -17.1441) (-6.9803, -17.1562) (-6.9794, -17.1682) (-6.9784, -17.1803) (-6.9775, -17.1925) (-6.9765, -17.2047) (-6.9755, -17.2169) (-6.9745, -17.2291) (-6.9735, -17.2414) (-6.9724, -17.2537) (-6.9713, -17.266) (-6.9702, -17.2784) (-6.9691, -17.2908) (-6.968, -17.3032) (-6.9669, -17.3157) (-6.9657, -17.3282) (-6.9645, -17.3407) (-6.9633, -17.3533) (-6.9621, -17.3659) (-6.9608, -17.3785) (-6.9596, -17.3912) (-6.9583, -17.4039) (-6.957, -17.4166) (-6.9556, -17.4293) (-6.9543, -17.4421) (-6.9529, -17.4549) (-6.9516, -17.4678) (-6.9501, -17.4806) (-6.9487, -17.4935) (-6.9473, -17.5065) (-6.9458, -17.5194) (-6.9443, -17.5324) (-6.9428, -17.5455) (-6.9413, -17.5585) (-6.9398, -17.5716) (-6.9382, -17.5847) (-6.9366, -17.5979) (-6.935, -17.611) (-6.9334, -17.6242) (-6.9317, -17.6375) (-6.9301, -17.6507) (-6.9284, -17.664) (-6.9267, -17.6773) (-6.925, -17.6907) (-6.9236, -17.7014) (-6.9225, -17.7094) (-6.9218, -17.7148) (-6.9214, -17.7174) knots 0 0 0 0 0 0 0.00416667 0.00833333 0.0125 0.01666667 0.02083333 0.025 0.02916667 0.03333333 0.0375 0.04166667 0.04583333 0.05 0.05416667 0.05833333 0.0625 0.06666667 0.07083333 0.075 0.07916667 0.08333333 0.0875 0.09166667 0.09583333 0.1 0.10416667 0.10833333 0.1125 0.11666667 0.12083333 0.125 0.12916667 0.13333333 0.1375 0.14166667 0.14583333 0.15 0.15416667 0.15833333 0.1625 0.16666667 0.17083333 0.175 0.17916667 0.18333333 0.1875 0.19166667 0.19583333 0.2 0.20416667 0.20833333 0.2125 0.21666667 0.22083333 0.225 0.22916667 0.23333333 0.2375 0.24166667 0.24583333 0.25 0.25416667 0.25833333 0.2625 0.26666667 0.27083333 0.275 0.27916667 0.28333333 0.2875 0.29166667 0.29583333 0.3 0.30416667 0.30833333 0.3125 0.31666667 0.32083333 0.325 0.32916667 0.33333333 0.3375 0.34166667 0.34583333 0.35 0.35416667 0.35833333 0.3625 0.36666667 0.37083333 0.375 0.37916667 0.38333333 0.3875 0.39166667 0.39583333 0.4 0.40416667 0.40833333 0.4125 0.41666667 0.42083333 0.425 0.42916667 0.43333333 0.4375 0.44166667 0.44583333 0.45 0.45416667 0.45833333 0.4625 0.46666667 0.47083333 0.475 0.47916667 0.48333333 0.4875 0.49166667 0.49583333 0.5 0.50416667 0.50833333 0.5125 0.51666667 0.52083333 0.525 0.52916667 0.53333333 0.5375 0.54166667 0.54583333 0.55 0.55416667 0.55833333 0.5625 0.56666667 0.57083333 0.575 0.57916667 0.58333333 0.5875 0.59166667 0.59583333 0.6 0.60416667 0.60833333 0.6125 0.61666667 0.62083333 0.625 0.62916667 0.63333333 0.6375 0.64166667 0.64583333 0.65 0.65416667 0.65833333 0.6625 0.66666667 0.67083333 0.675 0.67916667 0.68333333 0.6875 0.69166667 0.69583333 0.7 0.70416667 0.70833333 0.7125 0.71666667 0.72083333 0.725 0.72916667 0.73333333 0.7375 0.74166667 0.74583333 0.75 0.75416667 0.75833333 0.7625 0.76666667 0.77083333 0.775 0.77916667 0.78333333 0.7875 0.79166667 0.79583333 0.8 0.80416667 0.80833333 0.8125 0.81666667 0.82083333 0.825 0.82916667 0.83333333 0.8375 0.84166667 0.84583333 0.85 0.85416667 0.85833333 0.8625 0.86666667 0.87083333 0.875 0.87916667 0.88333333 0.8875 0.89166667 0.89583333 0.9 0.90416667 0.90833333 0.9125 0.91666667 0.92083333 0.925 0.92916667 0.93333333 0.9375 0.94166667 0.94583333 0.95 0.95416667 0.95833333 0.9625 0.96666667 0.97083333 0.975 0.97916667 0.98333333 0.9875 0.99166667 0.99583333 1 1 1 1 1 1
  arc A43 (-6.9214, -17.7174) -> (-5.9675, -17.9202) centre (0, 12.5) ccw
  spline S35 degree 5 poles (-5.9675, -17.9202) (-5.9661, -17.9179) (-5.9633, -17.9133) (-5.959, -17.9064) (-5.9534, -17.8972) (-5.9464, -17.8857) (-5.9394, -17.8742) (-5.9325, -17.8628) (-5.9255, -17.8513) (-5.9187, -17.8399) (-5.9118, -17.8285) (-5.905, -17.8171) (-5.8982, -17.8058) (-5.8914, -17.7944) (-5.8847, -17.7831) (-5.878, -17.7718) (-5.8713, -17.7605) (-5.8647, -17.7492) (-5.8581, -17.738) (-5.8515, -17.7268) (-5.8449, -17.7156) (-5.8384, -17.7044) (-5.8319, -17.6932) (-5.8255, -17.6821) (-5.8191, -17.6709) (-5.8127, -17.6598) (-5.8063, -17.6487) (-5.8, -17.6377) (-5.7937, -17.6266) (-5.7874, -17.6156) (-5.7811, -17.6046) (-5.7749, -17.5936) (-5.7688, -17.5826) (-5.7626, -17.5717) (-5.7565, -17.5608) (-5.7504, -17.5499) (-5.7443, -17.539) (-5.7383, -17.5281) (-5.7323, -17.5173) (-5.7263, -17.5065) (-5.7204, -17.4957) (-5.7145, -17.4849) (-5.7086, -17.4742) (-5.7028, -17.4634) (-5.697, -17.4527) (-5.6912, -17.4421) (-5.6854, -17.4314) (-5.6797, -17.4208) (-5.674, -17.4102) (-5.6683, -17.3996) (-5.6627, -17.389) (-5.6571, -17.3785) (-5.6515, -17.368) (-5.646, -17.3575) (-5.6405, -17.347) (-5.635, -17.3366) (-5.6296, -17.3262) (-5.6242, -17.3158) (-5.6188, -17.3054) (-5.6134, -17.2951) (-5.6081, -17.2847) (-5.6028, -17.2745) (-5.5975, -17.2642) (-5.5923, -17.254) (-5.5871, -17.2437) (-5.5819, -17.2336) (-5.5768, -17.2234) (-5.5717, -17.2133) (-5.5666, -17.2032) (-5.5615, -17.1931) (-5.5565, -17.183) (-5.5515, -17.173) (-5.5466, -17.163) (-5.5416, -17.153) (-5.5367, -17.1431) (-5.5319, -17.1332) (-5.527, -17.1233) (-5.5222, -17.1134) (-5.5175, -17.1036) (-5.5127, -17.0938) (-5.508, -17.084) (-5.5033, -17.0743) (-5.4987, -17.0646) (-5.494, -17.0549) (-5.4895, -17.0452) (-5.4849, -17.0356) (-5.4804, -17.026) (-5.4759, -17.0165) (-5.4714, -17.0069) (-5.467, -16.9974) (-5.4625, -16.9879) (-5.4582, -16.9785) (-5.4538, -16.9691) (-5.4495, -16.9597) (-5.4452, -16.9504) (-5.441, -16.941) (-5.4367, -16.9318) (-5.4325, -16.9225) (-5.4284, -16.9133) (-5.4242, -16.9041) (-5.4201, -16.895) (-5.4161, -16.8858) (-5.412, -16.8767) (-5.408, -16.8677) (-5.404, -16.8587) (-5.4001, -16.8497) (-5.3961, -16.8407) (-5.3922, -16.8318) (-5.3884, -16.8229) (-5.3846, -16.8141) (-5.3807, -16.8053) (-5.377, -16.7965) (-5.3732, -16.7878) (-5.3695, -16.779) (-5.3658, -16.7704) (-5.3622, -16.7617) (-5.3586, -16.7531) (-5.355, -16.7446) (-5.3514, -16.7361) (-5.3479, -16.7276) (-5.3444, -16.7191) (-5.3409, -16.7107) (-5.3375, -16.7023) (-5.3341, -16.694) (-5.3307, -16.6857) (-5.3273, -16.6775) (-5.324, -16.6692) (-5.3207, -16.6611) (-5.3175, -16.6529) (-5.3143, -16.6448) (-5.3111, -16.6368) (-5.3079, -16.6288) (-5.3047, -16.6208) (-5.3016, -16.6129) (-5.2986, -16.605) (-5.2955, -16.5971) (-5.2925, -16.5893) (-5.2895, -16.5815) (-5.2865, -16.5738) (-5.2836, -16.5661) (-5.2807, -16.5585) (-5.2778, -16.5509) (-5.275, -16.5433) (-5.2722, -16.5358) (-5.2694, -16.5284) (-5.2666, -16.521) (-5.2639, -16.5136) (-5.2612, -16.5063) (-5.2586, -16.499) (-5.2559, -16.4918) (-5.2533, -16.4846) (-5.2508, -16.4774) (-5.2482, -16.4703) (-5.2457, -16.4633) (-5.2432, -16.4563) (-5.2408, -16.4493) (-5.2383, -16.4424) (-5.2359, -16.4356) (-5.2336, -16.4288) (-5.2312, -16.422) (-5.2289, -16.4153) (-5.2266, -16.4087) (-5.2244, -16.4021) (-5.2222, -16.3955) (-5.22, -16.389) (-5.2178, -16.3826) (-5.2157, -16.3762) (-5.2136, -16.3699) (-5.2115, -16.3636) (-5.2094, -16.3573) (-5.2074, -16.3512) (-5.2054, -16.3451) (-5.2035, -16.339) (-5.2015, -16.333) (-5.1996, -16.327) (-5.1978, -16.3211) (-5.1959, -16.3153) (-5.1941, -16.3095) (-5.1923, -16.3038) (-5.1905, -16.2981) (-5.1888, -16.2925) (-5.1871, -16.2869) (-5.1854, -16.2815) (-5.1838, -16.276) (-5.1822, -16.2707) (-5.1806, -16.2654) (-5.179, -16.2601) (-5.1775, -16.2549) (-5.176, -16.2498) (-5.1745, -16.2448) (-5.173, -16.2398) (-5.1716, -16.2349) (-5.1702, -16.23) (-5.1689, -16.2252) (-5.1675, -16.2205) (-5.1662, -16.2158) (-5.1649, -16.2112) (-5.1637, -16.2067) (-5.1625, -16.2023) (-5.1613, -16.1979) (-5.1601, -16.1936) (-5.1589, -16.1893) (-5.1578, -16.1852) (-5.1567, -16.1811) (-5.1557, -16.1771) (-5.1546, -16.1731) (-5.1536, -16.1693) (-5.1527, -16.1655) (-5.1517, -16.1617) (-5.1508, -16.1581) (-5.1499, -16.1545) (-5.149, -16.1511) (-5.1481, -16.1477) (-5.1473, -16.1443) (-5.1465, -16.1411) (-5.1458, -16.1379) (-5.145, -16.1349) (-5.1443, -16.1319) (-5.1436, -16.129) (-5.143, -16.1262) (-5.1423, -16.1234) (-5.1417, -16.1208) (-5.1411, -16.1182) (-5.1406, -16.1158) (-5.14, -16.1134) (-5.1395, -16.1111) (-5.139, -16.1089) (-5.1386, -16.1069) (-5.1381, -16.1049) (-5.1377, -16.103) (-5.1374, -16.1012) (-5.137, -16.0995) (-5.1367, -16.0979) (-5.1363, -16.0964) (-5.1361, -16.095) (-5.1358, -16.0937) (-5.1356, -16.0925) (-5.1354, -16.0915) (-5.1352, -16.0905) (-5.135, -16.0896) (-5.1349, -16.0889) (-5.1348, -16.0884) (-5.1347, -16.0881) (-5.1347, -16.0879) (-5.1346, -16.0878) knots -1 -1 -1 -1 -1 -1 -0.99583333 -0.99166667 -0.9875 -0.98333333 -0.97916667 -0.975 -0.97083333 -0.96666667 -0.9625 -0.95833333 -0.95416667 -0.95 -0.94583333 -0.94166667 -0.9375 -0.93333333 -0.92916667 -0.925 -0.92083333 -0.91666667 -0.9125 -0.90833333 -0.90416667 -0.9 -0.89583333 -0.89166667 -0.8875 -0.88333333 -0.87916667 -0.875 -0.87083333 -0.86666667 -0.8625 -0.85833333 -0.85416667 -0.85 -0.84583333 -0.84166667 -0.8375 -0.83333333 -0.82916667 -0.825 -0.82083333 -0.81666667 -0.8125 -0.80833333 -0.80416667 -0.8 -0.79583333 -0.79166667 -0.7875 -0.78333333 -0.77916667 -0.775 -0.77083333 -0.76666667 -0.7625 -0.75833333 -0.75416667 -0.75 -0.74583333 -0.74166667 -0.7375 -0.73333333 -0.72916667 -0.725 -0.72083333 -0.71666667 -0.7125 -0.70833333 -0.70416667 -0.7 -0.69583333 -0.69166667 -0.6875 -0.68333333 -0.67916667 -0.675 -0.67083333 -0.66666667 -0.6625 -0.65833333 -0.65416667 -0.65 -0.64583333 -0.64166667 -0.6375 -0.63333333 -0.62916667 -0.625 -0.62083333 -0.61666667 -0.6125 -0.60833333 -0.60416667 -0.6 -0.59583333 -0.59166667 -0.5875 -0.58333333 -0.57916667 -0.575 -0.57083333 -0.56666667 -0.5625 -0.55833333 -0.55416667 -0.55 -0.54583333 -0.54166667 -0.5375 -0.53333333 -0.52916667 -0.525 -0.52083333 -0.51666667 -0.5125 -0.50833333 -0.50416667 -0.5 -0.49583333 -0.49166667 -0.4875 -0.48333333 -0.47916667 -0.475 -0.47083333 -0.46666667 -0.4625 -0.45833333 -0.45416667 -0.45 -0.44583333 -0.44166667 -0.4375 -0.43333333 -0.42916667 -0.425 -0.42083333 -0.41666667 -0.4125 -0.40833333 -0.40416667 -0.4 -0.39583333 -0.39166667 -0.3875 -0.38333333 -0.37916667 -0.375 -0.37083333 -0.36666667 -0.3625 -0.35833333 -0.35416667 -0.35 -0.34583333 -0.34166667 -0.3375 -0.33333333 -0.32916667 -0.325 -0.32083333 -0.31666667 -0.3125 -0.30833333 -0.30416667 -0.3 -0.29583333 -0.29166667 -0.2875 -0.28333333 -0.27916667 -0.275 -0.27083333 -0.26666667 -0.2625 -0.25833333 -0.25416667 -0.25 -0.24583333 -0.24166667 -0.2375 -0.23333333 -0.22916667 -0.225 -0.22083333 -0.21666667 -0.2125 -0.20833333 -0.20416667 -0.2 -0.19583333 -0.19166667 -0.1875 -0.18333333 -0.17916667 -0.175 -0.17083333 -0.16666667 -0.1625 -0.15833333 -0.15416667 -0.15 -0.14583333 -0.14166667 -0.1375 -0.13333333 -0.12916667 -0.125 -0.12083333 -0.11666667 -0.1125 -0.10833333 -0.10416667 -0.1 -0.09583333 -0.09166667 -0.0875 -0.08333333 -0.07916667 -0.075 -0.07083333 -0.06666667 -0.0625 -0.05833333 -0.05416667 -0.05 -0.04583333 -0.04166667 -0.0375 -0.03333333 -0.02916667 -0.025 -0.02083333 -0.01666667 -0.0125 -0.00833333 -0.00416667 0 0 0 0 0 0
  line L71 (-5.1346, -16.0878) -> (-5.1345, -16.087)
  line L72 (-5.1345, -16.087) -> (-5.0824, -15.7972)
  arc A44 (-5.0824, -15.7972) -> (-3.9106, -15.9828) centre (0, 12.5) ccw
  line L73 (-3.9106, -15.9828) -> (-3.9507, -16.2745)
  line L74 (-3.9507, -16.2745) -> (-3.9508, -16.2753)